Autodesk Inventor part; units mm, degrees
(part 2 of 3)
  line L934 (-2.3825, 17.3276) -> (-2.1489, 17.5795)
  line L935 (-2.1489, 17.5795) -> (-1.9408, 17.8528)
  line L936 (-1.9408, 17.8528) -> (-1.76, 18.1449)
  line L937 (-1.76, 18.1449) -> (-1.6083, 18.4531)
  line L938 (-2.6725, 3.5253) -> (-2.5898, 3.5474)
  line L939 (-16.7895, -16.1624) -> (-16.4169, -16.535)
  line L940 (-15.9078, -14.6352) -> (-16.4089, -14.7796)
  line L941 (15.6533, -16.6714) -> (16.1624, -16.535)
  line L942 (15.502, -16.5103) -> (16.0062, -16.3752)
  line L943 (-2.5898, 3.8338) -> (-2.6725, 3.856)
  line L944 (-2.5648, 3.7968) -> (-2.6467, 3.8187)
  line L945 (-15.0316, -16.1569) -> (-14.8897, -15.6533)
  line L946 (15.1443, -16.535) -> (15.6533, -16.6714)
  line L947 (14.9979, -16.3752) -> (15.502, -16.5103)
  line L948 (14.7716, -16.1624) -> (14.9979, -16.3752)
  line L949 (-12.7709, 17.5782) -> (-12.8535, 17.6003)
  line L950 (-12.6921, 17.4203) -> (-12.7293, 17.4302)
  line L951 (11.4696, 12.9362) -> (11.4091, 12.9967)
  line L952 (4.4542, 16.535) -> (4.0815, 16.1624)
  line L953 (-14.1262, 17.2697) -> (-14.0435, 17.2918)
  line L954 (-2.5293, 3.6079) -> (-2.4935, 3.6943)
  line L955 (-15.3161, -0.4931) -> (-15.3988, -0.471)
  line L956 (-2.7552, 3.5474) -> (-2.6725, 3.5253)
  line L957 (-11.6922, 17.5177) -> (-11.7528, 17.5782)
  line L958 (-12.8535, 17.6003) -> (-12.9362, 17.5782)
  line L959 (-12.7293, 17.4302) -> (-12.8112, 17.4083)
  line L960 (-14.0435, 17.2918) -> (-13.983, 17.3523)
  line L961 (16.535, -16.1624) -> (16.6714, -15.6533)
  line L962 (16.3752, -16.0062) -> (16.5103, -15.502)
  line L963 (16.1624, -16.535) -> (16.535, -16.1624)
  line L964 (16.0062, -16.3752) -> (16.3752, -16.0062)
  line L965 (-16.051, 13.0254) -> (-15.9905, 12.9649)
  line L966 (16.5103, -15.502) -> (16.3752, -14.9979)
  line L967 (10.4801, 13.5058) -> (10.4196, 13.4453)
  line L968 (-12.9362, 17.5782) -> (-12.9967, 17.5177)
  line L969 (-8.8703, 17.435) -> (-8.8925, 17.5177)
  line L970 (16.3752, -14.9979) -> (16.1624, -14.7716)
  line L971 (16.6714, -15.6533) -> (16.535, -15.1443)
  line L972 (-1.0022, 5.6442) -> (-0.985, 5.7255)
  line L973 (-9.1183, 17.5782) -> (-9.1788, 17.5177)
  line L974 (-9.0302, 17.4083) -> (-9.0901, 17.3484)
  line L975 (10.706, 13.2799) -> (10.7282, 13.3626)
  line L976 (14.7784, 2.3353) -> (14.8006, 2.418)
  line L977 (14.6356, 2.3128) -> (14.6575, 2.3946)
  line L978 (10.5628, 13.5279) -> (10.4801, 13.5058)
  line L979 (-13.983, 17.5177) -> (-14.0435, 17.5782)
  line L980 (5.4723, 14.7716) -> (5.8449, 15.1443)
  line L981 (4.9632, 14.6352) -> (5.4723, 14.7716)
  line L982 (16.1699, -9.0744) -> (16.1502, -9.0008)
  line L983 (3.9451, 15.6533) -> (4.0815, 15.1443)
  line L984 (11.1545, -2.0203) -> (11.0719, -1.9981)
  line L985 (4.4542, 14.7716) -> (4.9632, 14.6352)
  line L986 (13.2334, -15.1616) -> (13.3153, -15.1397)
  line L987 (-13.0189, 17.435) -> (-12.9967, 17.3523)
  line L988 (-11.7528, 17.2918) -> (-11.6922, 17.3523)
  line L989 (10.4196, 13.4453) -> (10.3975, 13.3626)
  line L990 (-17.5782, 6.6623) -> (-17.5177, 6.6017)
  line L991 (-8.953, 17.5782) -> (-9.0357, 17.6003)
  line L992 (-8.8767, 17.411) -> (-8.9483, 17.4302)
  line L993 (-2.7885, 3.5731) -> (-2.7552, 3.5474)
  line L994 (16.1624, -14.7716) -> (15.6533, -14.6352)
  line L995 (-11.8354, 17.6003) -> (-11.9181, 17.5782)
  line L996 (-11.721, 17.4302) -> (-11.8029, 17.4083)
  line L997 (5.8449, 16.1624) -> (5.4723, 16.535)
  line L998 (4.0815, 15.1443) -> (4.4542, 14.7716)
  line L999 (5.9813, 15.6533) -> (5.8449, 16.1624)
  line L1000 (-17.2697, 9.2902) -> (-17.2918, 9.3729)
  line L1001 (5.9235, 15.502) -> (5.7885, 16.0062)
  line L1002 (14.7179, 2.2748) -> (14.7784, 2.3353)
  line L1003 (14.5881, 2.2653) -> (14.6356, 2.3128)
  line L1004 (-11.8354, 17.2697) -> (-11.7528, 17.2918)
  line L1005 (-1.0627, 5.5836) -> (-1.0022, 5.6442)
  line L1006 (-17.2918, 9.3729) -> (-17.3523, 9.4334)
  line L1007 (4.9632, 16.6714) -> (4.4542, 16.535)
  line L1008 (15.6533, -14.6352) -> (15.1443, -14.7716)
  line L1009 (-17.6003, 6.7449) -> (-17.5782, 6.6623)
  line L1010 (-1.1454, 5.5615) -> (-1.0627, 5.5836)
  line L1011 (15.1443, -14.7716) -> (14.7716, -15.1443)
  line L1012 (14.7716, -15.1443) -> (14.6352, -15.6533)
  line L1013 (-17.435, 6.9103) -> (-17.5177, 6.8881)
  line L1014 (-9.0357, 17.6003) -> (-9.1183, 17.5782)
  line L1015 (-8.9483, 17.4302) -> (-9.0302, 17.4083)
  line L1016 (-1.228, 5.5836) -> (-1.1454, 5.5615)
  line L1017 (-14.6352, 15.6533) -> (-14.7716, 16.1624)
  line L1018 (-16.1624, 14.7716) -> (-15.6533, 14.6352)
  line L1019 (-16.6714, 15.6533) -> (-16.535, 15.1443)
  line L1020 (-16.535, 16.1624) -> (-16.6714, 15.6533)
  line L1021 (-16.1624, 16.535) -> (-16.535, 16.1624)
  line L1022 (-15.6533, 16.6714) -> (-16.1624, 16.535)
  line L1023 (-15.9078, -16.6714) -> (-15.3988, -16.535)
  line L1024 (-16.4169, -16.535) -> (-15.9078, -16.6714)
  line L1025 (-16.9259, -15.6533) -> (-16.7895, -16.1624)
  line L1026 (-15.3988, -14.7716) -> (-15.9078, -14.6352)
  line L1027 (16.026, -3.4361) -> (16.1624, -2.927)
  line L1028 (15.6533, -3.8087) -> (16.026, -3.4361)
  line L1029 (15.1443, -3.9451) -> (15.6533, -3.8087)
  line L1030 (14.1262, -2.927) -> (14.2626, -3.4361)
  line L1031 (14.2626, -2.418) -> (14.1262, -2.927)
  line L1032 (14.6352, -2.0453) -> (14.2626, -2.418)
  line L1033 (15.6533, -2.0453) -> (15.1443, -1.9089)
  line L1034 (16.026, -2.418) -> (15.6533, -2.0453)
  line L1035 (-13.1081, 15.017) -> (-13.1763, 15.2715)
  line L1036 (-13.1763, 14.7625) -> (-13.1081, 15.017)
  line L1037 (-13.3626, 14.5762) -> (-13.1763, 14.7625)
  line L1038 (-13.6171, 14.508) -> (-13.3626, 14.5762)
  line L1039 (-13.8716, 14.5762) -> (-13.6171, 14.508)
  line L1040 (-14.1262, 15.017) -> (-14.058, 14.7625)
  line L1041 (-14.058, 15.2715) -> (-14.1262, 15.017)
  line L1042 (-13.8716, 15.4579) -> (-14.058, 15.2715)
  line L1043 (-13.6171, 15.5261) -> (-13.8716, 15.4579)
  line L1044 (-13.3626, 15.4579) -> (-13.6171, 15.5261)
  line L1045 (-8.0858, 15.7806) -> (-8.0176, 16.0351)
  line L1046 (-8.2721, 15.5943) -> (-8.0858, 15.7806)
  line L1047 (-8.5266, 15.5261) -> (-8.2721, 15.5943)
  line L1048 (-8.7811, 15.5943) -> (-8.5266, 15.5261)
  line L1049 (-9.0357, 16.0351) -> (-8.9675, 15.7806)
  line L1050 (-8.9675, 16.2896) -> (-9.0357, 16.0351)
  line L1051 (-8.7811, 16.476) -> (-8.9675, 16.2896)
  line L1052 (-8.5266, 16.5442) -> (-8.7811, 16.476)
  line L1053 (-8.2721, 16.476) -> (-8.5266, 16.5442)
  line L1054 (-8.0858, 16.2896) -> (-8.2721, 16.476)
  line L1055 (-8.0858, 13.7444) -> (-8.0176, 13.9989)
  line L1056 (-8.2721, 13.5581) -> (-8.0858, 13.7444)
  line L1057 (-8.7811, 13.5581) -> (-8.5266, 13.4899)
  line L1058 (-8.7811, 14.4398) -> (-8.9675, 14.2534)
  line L1059 (-8.0858, 14.2534) -> (-8.2721, 14.4398)
  line L1060 (-12.5163, 12.9649) -> (-12.4558, 13.0254)
  line L1061 (-12.599, 12.9427) -> (-12.5163, 12.9649)
  line L1062 (-12.7422, 13.0254) -> (-12.6817, 12.9649)
  line L1063 (-12.7644, 13.1081) -> (-12.7422, 13.0254)
  line L1064 (-12.7422, 13.1907) -> (-12.7644, 13.1081)
  line L1065 (-12.6817, 13.2513) -> (-12.7422, 13.1907)
  line L1066 (-12.599, 13.2734) -> (-12.6817, 13.2513)
  line L1067 (-12.5163, 13.2513) -> (-12.599, 13.2734)
  line L1068 (-12.4558, 13.1907) -> (-12.5163, 13.2513)
  line L1069 (-1.228, 5.87) -> (-1.2886, 5.8095)
  line L1070 (-1.1454, 5.8922) -> (-1.228, 5.87)
  line L1071 (-1.0627, 5.87) -> (-1.1454, 5.8922)
  line L1072 (-9.0357, 17.2697) -> (-8.953, 17.2918)
  line L1073 (-9.1183, 17.2918) -> (-9.0357, 17.2697)
  line L1074 (-9.1788, 17.3523) -> (-9.1183, 17.2918)
  line L1075 (11.4917, 12.8535) -> (11.4696, 12.9362)
  line L1076 (11.4091, 12.7103) -> (11.4696, 12.7709)
  line L1077 (11.2437, 12.7103) -> (11.3264, 12.6882)
  line L1078 (11.1832, 12.7709) -> (11.2437, 12.7103)
  line L1079 (11.161, 12.8535) -> (11.1832, 12.7709)
  line L1080 (11.2437, 12.9967) -> (11.1832, 12.9362)
  line L1081 (11.3264, 13.0189) -> (11.2437, 12.9967)
  line L1082 (11.4091, 12.9967) -> (11.3264, 13.0189)
  line L1083 (-11.6922, 17.3523) -> (-11.6701, 17.435)
  line L1084 (-11.9786, 17.5177) -> (-12.0008, 17.435)
  line L1085 (-11.9181, 17.5782) -> (-11.9786, 17.5177)
  line L1086 (10.7282, 13.3626) -> (10.706, 13.4453)
  line L1087 (10.6455, 13.2194) -> (10.706, 13.2799)
  line L1088 (10.4801, 13.2194) -> (10.5628, 13.1972)
  line L1089 (10.4196, 13.2799) -> (10.4801, 13.2194)
  line L1090 (10.3975, 13.3626) -> (10.4196, 13.2799)
  line L1091 (10.706, 13.4453) -> (10.6455, 13.5058)
  line L1092 (8.1829, 15.1443) -> (8.1607, 15.2269)
  line L1093 (8.1607, 15.0616) -> (8.1829, 15.1443)
  line L1094 (8.1002, 15.0011) -> (8.1607, 15.0616)
  line L1095 (8.0176, 14.9789) -> (8.1002, 15.0011)
  line L1096 (7.9349, 15.0011) -> (8.0176, 14.9789)
  line L1097 (7.8744, 15.0616) -> (7.9349, 15.0011)
  line L1098 (7.8522, 15.1443) -> (7.8744, 15.0616)
  line L1099 (7.8744, 15.2269) -> (7.8522, 15.1443)
  line L1100 (7.9349, 15.2875) -> (7.8744, 15.2269)
  line L1101 (8.0176, 15.3096) -> (7.9349, 15.2875)
  line L1102 (8.1002, 15.2875) -> (8.0176, 15.3096)
  line L1103 (8.1607, 15.2269) -> (8.1002, 15.2875)
  line L1104 (-1.2345, 16.4169) -> (-1.2567, 16.4996)
  line L1105 (-1.2477, 16.3432) -> (-1.2345, 16.4169)
  line L1106 (-1.3172, 16.2737) -> (-1.2477, 16.3432)
  line L1107 (-1.3999, 16.2516) -> (-1.3172, 16.2737)
  line L1108 (-1.4826, 16.2737) -> (-1.3999, 16.2516)
  line L1109 (-1.5431, 16.3342) -> (-1.4826, 16.2737)
  line L1110 (-1.5652, 16.4169) -> (-1.5431, 16.3342)
  line L1111 (-1.5431, 16.4996) -> (-1.5652, 16.4169)
  line L1112 (-1.4826, 16.5601) -> (-1.5431, 16.4996)
  line L1113 (-1.3999, 16.5822) -> (-1.4826, 16.5601)
  line L1114 (-1.3172, 16.5601) -> (-1.3999, 16.5822)
  line L1115 (-1.2567, 16.4996) -> (-1.3172, 16.5601)
  line L1116 (10.7282, 15.3988) -> (10.706, 15.4815)
  line L1117 (10.706, 15.4815) -> (10.6455, 15.542)
  line L1118 (14.546, -12.599) -> (14.5239, -12.5163)
  line L1119 (14.5239, -12.6817) -> (14.546, -12.599)
  line L1120 (14.4634, -12.7422) -> (14.5239, -12.6817)
  line L1121 (14.3807, -12.7644) -> (14.4634, -12.7422)
  line L1122 (14.298, -12.7422) -> (14.3807, -12.7644)
  line L1123 (14.2375, -12.6817) -> (14.298, -12.7422)
  line L1124 (14.2375, -12.5163) -> (14.2154, -12.599)
  line L1125 (14.298, -12.4558) -> (14.2375, -12.5163)
  line L1126 (14.3807, -12.4337) -> (14.298, -12.4558)
  line L1127 (14.4634, -12.4558) -> (14.3807, -12.4337)
  line L1128 (14.5239, -12.5163) -> (14.4634, -12.4558)
  line L1129 (6.6557, -17.435) -> (6.6336, -17.3523)
  line L1130 (6.6336, -17.5177) -> (6.6557, -17.435)
  line L1131 (6.5731, -17.5782) -> (6.6336, -17.5177)
  line L1132 (6.4904, -17.6003) -> (6.5731, -17.5782)
  line L1133 (6.4077, -17.5782) -> (6.4904, -17.6003)
  line L1134 (6.3472, -17.5177) -> (6.4077, -17.5782)
  line L1135 (6.3251, -17.435) -> (6.3472, -17.5177)
  line L1136 (6.4077, -17.2918) -> (6.3472, -17.3523)
  line L1137 (6.4904, -17.2697) -> (6.4077, -17.2918)
  line L1138 (6.5731, -17.2918) -> (6.4904, -17.2697)
  line L1139 (6.6336, -17.3523) -> (6.5731, -17.2918)
  line L1140 (0.0381, -17.435) -> (0.0159, -17.3523)
  line L1141 (0.0159, -17.5177) -> (0.0381, -17.435)
  line L1142 (-0.0446, -17.5782) -> (0.0159, -17.5177)
  line L1143 (-0.1273, -17.6003) -> (-0.0446, -17.5782)
  line L1144 (-0.2099, -17.5782) -> (-0.1273, -17.6003)
  line L1145 (-0.2705, -17.5177) -> (-0.2099, -17.5782)
  line L1146 (-0.2099, -17.2918) -> (-0.2705, -17.3523)
  line L1147 (-0.1273, -17.2697) -> (-0.2099, -17.2918)
  line L1148 (-0.0446, -17.2918) -> (-0.1273, -17.2697)
  line L1149 (0.0159, -17.3523) -> (-0.0446, -17.2918)
  line L1150 (-5.8382, -15.736) -> (-5.816, -15.6533)
  line L1151 (-5.8987, -15.7965) -> (-5.8382, -15.736)
  line L1152 (-5.9813, -15.8187) -> (-5.8987, -15.7965)
  line L1153 (-6.064, -15.7965) -> (-5.9813, -15.8187)
  line L1154 (-6.1245, -15.736) -> (-6.064, -15.7965)
  line L1155 (-6.1467, -15.6533) -> (-6.1245, -15.736)
  line L1156 (-6.1245, -15.5706) -> (-6.1467, -15.6533)
  line L1157 (-5.9813, -15.488) -> (-6.064, -15.5101)
  line L1158 (-5.8987, -15.5101) -> (-5.9813, -15.488)
  line L1159 (-5.8382, -15.5706) -> (-5.8987, -15.5101)
  line L1160 (-8.8703, -14.8897) -> (-8.8925, -14.8071)
  line L1161 (-8.8925, -14.9724) -> (-8.8703, -14.8897)
  line L1162 (-8.953, -15.0329) -> (-8.8925, -14.9724)
  line L1163 (-9.0357, -15.0551) -> (-8.953, -15.0329)
  line L1164 (-9.1183, -15.0329) -> (-9.0357, -15.0551)
  line L1165 (-9.1788, -14.9724) -> (-9.1183, -15.0329)
  line L1166 (-9.201, -14.8897) -> (-9.1788, -14.9724)
  line L1167 (-9.1788, -14.8071) -> (-9.201, -14.8897)
  line L1168 (-9.1183, -14.7466) -> (-9.1788, -14.8071)
  line L1169 (-9.0357, -14.7244) -> (-9.1183, -14.7466)
  line L1170 (-8.953, -14.7466) -> (-9.0357, -14.7244)
  line L1171 (-8.8925, -14.8071) -> (-8.953, -14.7466)
  line L1172 (-11.6701, -14.8897) -> (-11.6922, -14.8071)
  line L1173 (-11.6922, -14.9724) -> (-11.6701, -14.8897)
  line L1174 (-11.7528, -15.0329) -> (-11.6922, -14.9724)
  line L1175 (-11.8354, -15.0551) -> (-11.7528, -15.0329)
  line L1176 (-11.9181, -15.0329) -> (-11.8354, -15.0551)
  line L1177 (-11.9786, -14.9724) -> (-11.9181, -15.0329)
  line L1178 (-12.0008, -14.8897) -> (-11.9786, -14.9724)
  line L1179 (-11.9786, -14.8071) -> (-12.0008, -14.8897)
  line L1180 (-11.9181, -14.7466) -> (-11.9786, -14.8071)
  line L1181 (-11.7528, -14.7466) -> (-11.8354, -14.7244)
  line L1182 (-11.6922, -14.8071) -> (-11.7528, -14.7466)
  line L1183 (-13.4518, -15.9078) -> (-13.4739, -15.8252)
  line L1184 (-13.4739, -15.9905) -> (-13.4518, -15.9078)
  line L1185 (-13.5344, -16.051) -> (-13.4739, -15.9905)
  line L1186 (-13.6171, -16.0732) -> (-13.5344, -16.051)
  line L1187 (-13.6998, -16.051) -> (-13.6171, -16.0732)
  line L1188 (-13.7603, -15.9905) -> (-13.6998, -16.051)
  line L1189 (-13.7825, -15.9078) -> (-13.7603, -15.9905)
  line L1190 (-13.7603, -15.8252) -> (-13.7825, -15.9078)
  line L1191 (-13.6998, -15.7647) -> (-13.7603, -15.8252)
  line L1192 (-13.5344, -15.7647) -> (-13.6171, -15.7425)
  line L1193 (-13.4739, -15.8252) -> (-13.5344, -15.7647)
  line L1194 (-15.0011, -17.3904) -> (-14.9789, -17.3077)
  line L1195 (-15.0616, -17.4509) -> (-15.0011, -17.3904)
  line L1196 (-15.1443, -17.4731) -> (-15.0616, -17.4509)
  line L1197 (-15.2269, -17.4509) -> (-15.1443, -17.4731)
  line L1198 (-15.2875, -17.3904) -> (-15.2269, -17.4509)
  line L1199 (-15.3096, -17.3077) -> (-15.2875, -17.3904)
  line L1200 (-15.2875, -17.2251) -> (-15.3096, -17.3077)
  line L1201 (-15.2269, -17.1645) -> (-15.2875, -17.2251)
  line L1202 (-15.1443, -17.1424) -> (-15.2269, -17.1645)
  line L1203 (-15.0616, -17.1645) -> (-15.1443, -17.1424)
  line L1204 (-15.0011, -17.2251) -> (-15.0616, -17.1645)
  line L1205 (-17.2697, -14.7625) -> (-17.2918, -14.6798)
  line L1206 (-17.3523, -14.9057) -> (-17.2918, -14.8452)
  line L1207 (-17.435, -14.9278) -> (-17.3523, -14.9057)
  line L1208 (-17.5177, -14.9057) -> (-17.435, -14.9278)
  line L1209 (-17.5782, -14.8452) -> (-17.5177, -14.9057)
  line L1210 (-17.6003, -14.7625) -> (-17.5782, -14.8452)
  line L1211 (-17.5782, -14.6798) -> (-17.6003, -14.7625)
  line L1212 (-17.5177, -14.6193) -> (-17.5782, -14.6798)
  line L1213 (-17.435, -14.5971) -> (-17.5177, -14.6193)
  line L1214 (-17.3523, -14.6193) -> (-17.435, -14.5971)
  line L1215 (-17.2918, -14.6798) -> (-17.3523, -14.6193)
  line L1216 (-15.488, -13.3626) -> (-15.5101, -13.2799)
  line L1217 (-15.5706, -13.5058) -> (-15.5101, -13.4453)
  line L1218 (-15.6533, -13.5279) -> (-15.5706, -13.5058)
  line L1219 (-15.736, -13.5058) -> (-15.6533, -13.5279)
  line L1220 (-15.7965, -13.4453) -> (-15.736, -13.5058)
  line L1221 (-15.8187, -13.3626) -> (-15.7965, -13.4453)
  line L1222 (-15.7965, -13.2799) -> (-15.8187, -13.3626)
  line L1223 (-15.736, -13.2194) -> (-15.7965, -13.2799)
  line L1224 (-15.6533, -13.1972) -> (-15.736, -13.2194)
  line L1225 (-15.5706, -13.2194) -> (-15.6533, -13.1972)
  line L1226 (-15.5101, -13.2799) -> (-15.5706, -13.2194)
  line L1227 (-14.9789, -11.5809) -> (-15.0011, -11.4982)
  line L1228 (-15.0616, -11.7241) -> (-15.0011, -11.6636)
  line L1229 (-15.1443, -11.7463) -> (-15.0616, -11.7241)
  line L1230 (-15.2269, -11.7241) -> (-15.1443, -11.7463)
  line L1231 (-15.2875, -11.6636) -> (-15.2269, -11.7241)
  line L1232 (-15.3096, -11.5809) -> (-15.2875, -11.6636)
  line L1233 (-15.2875, -11.4982) -> (-15.3096, -11.5809)
  line L1234 (-15.2269, -11.4377) -> (-15.2875, -11.4982)
  line L1235 (-15.1443, -11.4156) -> (-15.2269, -11.4377)
  line L1236 (-15.0616, -11.4377) -> (-15.1443, -11.4156)
  line L1237 (-15.0011, -11.4982) -> (-15.0616, -11.4377)
  line L1238 (-14.7244, -8.7811) -> (-14.7466, -8.6985)
  line L1239 (-14.7466, -8.8638) -> (-14.7244, -8.7811)
  line L1240 (-14.8071, -8.9243) -> (-14.7466, -8.8638)
  line L1241 (-14.8897, -8.9465) -> (-14.8071, -8.9243)
  line L1242 (-14.9724, -8.9243) -> (-14.8897, -8.9465)
  line L1243 (-15.0329, -8.8638) -> (-14.9724, -8.9243)
  line L1244 (-15.0551, -8.7811) -> (-15.0329, -8.8638)
  line L1245 (-15.0329, -8.6985) -> (-15.0551, -8.7811)
  line L1246 (-14.9724, -8.6379) -> (-15.0329, -8.6985)
  line L1247 (-14.8897, -8.6158) -> (-14.9724, -8.6379)
  line L1248 (-14.8071, -8.6379) -> (-14.8897, -8.6158)
  line L1249 (-14.7466, -8.6985) -> (-14.8071, -8.6379)
  line L1250 (-15.488, -6.2359) -> (-15.5101, -6.1532)
  line L1251 (-15.5101, -6.3185) -> (-15.488, -6.2359)
  line L1252 (-15.5706, -6.3791) -> (-15.5101, -6.3185)
  line L1253 (-15.6533, -6.4012) -> (-15.5706, -6.3791)
  line L1254 (-15.736, -6.3791) -> (-15.6533, -6.4012)
  line L1255 (-15.7965, -6.3185) -> (-15.736, -6.3791)
  line L1256 (-15.8187, -6.2359) -> (-15.7965, -6.3185)
  line L1257 (-15.7965, -6.1532) -> (-15.8187, -6.2359)
  line L1258 (-15.736, -6.0927) -> (-15.7965, -6.1532)
  line L1259 (-15.6533, -6.0705) -> (-15.736, -6.0927)
  line L1260 (-15.5101, -6.1532) -> (-15.5706, -6.0927)
  line L1261 (-17.2697, -4.1997) -> (-17.2918, -4.117)
  line L1262 (-17.2918, -4.2823) -> (-17.2697, -4.1997)
  line L1263 (-17.435, -4.365) -> (-17.3523, -4.3429)
  line L1264 (-17.5177, -4.3429) -> (-17.435, -4.365)
  line L1265 (-17.5782, -4.2823) -> (-17.5177, -4.3429)
  line L1266 (-17.6003, -4.1997) -> (-17.5782, -4.2823)
  line L1267 (-17.5782, -4.117) -> (-17.6003, -4.1997)
  line L1268 (-17.5177, -4.0565) -> (-17.5782, -4.117)
  line L1269 (-17.435, -4.0343) -> (-17.5177, -4.0565)
  line L1270 (-17.2918, -4.117) -> (-17.3523, -4.0565)
  line L1271 (-17.2697, -1.6544) -> (-17.2918, -1.5717)
  line L1272 (-17.2918, -1.7371) -> (-17.2697, -1.6544)
  line L1273 (-17.3523, -1.7976) -> (-17.2918, -1.7371)
  line L1274 (-17.435, -1.8198) -> (-17.3523, -1.7976)
  line L1275 (-17.5177, -1.7976) -> (-17.435, -1.8198)
  line L1276 (-17.5782, -1.7371) -> (-17.5177, -1.7976)
  line L1277 (-17.6003, -1.6544) -> (-17.5782, -1.7371)
  line L1278 (-17.5782, -1.5717) -> (-17.6003, -1.6544)
  line L1279 (-17.5177, -1.5112) -> (-17.5782, -1.5717)
  line L1280 (-17.435, -1.4891) -> (-17.5177, -1.5112)
  line L1281 (-17.3523, -1.5112) -> (-17.435, -1.4891)
  line L1282 (-17.2918, -1.5717) -> (-17.3523, -1.5112)
  line L1283 (-17.2697, 0.8908) -> (-17.2918, 0.9735)
  line L1284 (-17.2918, 0.8082) -> (-17.2697, 0.8908)
  line L1285 (-17.3523, 0.7476) -> (-17.2918, 0.8082)
  line L1286 (-17.435, 0.7255) -> (-17.3523, 0.7476)
  line L1287 (-17.5177, 0.7476) -> (-17.435, 0.7255)
  line L1288 (-17.5782, 0.8082) -> (-17.5177, 0.7476)
  line L1289 (-17.6003, 0.8908) -> (-17.5782, 0.8082)
  line L1290 (-17.5782, 0.9735) -> (-17.6003, 0.8908)
  line L1291 (-17.5177, 1.034) -> (-17.5782, 0.9735)
  line L1292 (-17.435, 1.0562) -> (-17.5177, 1.034)
  line L1293 (-17.3523, 1.034) -> (-17.435, 1.0562)
  line L1294 (-17.2918, 0.9735) -> (-17.3523, 1.034)
  line L1295 (-17.2697, 3.6906) -> (-17.2918, 3.7733)
  line L1296 (-17.2918, 3.6079) -> (-17.2697, 3.6906)
  line L1297 (-17.3523, 3.5474) -> (-17.2918, 3.6079)
  line L1298 (-17.5177, 3.5474) -> (-17.435, 3.5253)
  line L1299 (-17.5782, 3.6079) -> (-17.5177, 3.5474)
  line L1300 (-17.6003, 3.6906) -> (-17.5782, 3.6079)
  line L1301 (-17.5782, 3.7733) -> (-17.6003, 3.6906)
  line L1302 (-17.5177, 3.8338) -> (-17.5782, 3.7733)
  line L1303 (-17.435, 3.856) -> (-17.5177, 3.8338)
  line L1304 (-17.3523, 3.8338) -> (-17.435, 3.856)
  line L1305 (-17.2697, 6.7449) -> (-17.2918, 6.8276)
  line L1306 (-17.2918, 6.6623) -> (-17.2697, 6.7449)
  line L1307 (-17.3523, 6.6017) -> (-17.2918, 6.6623)
  line L1308 (-17.5177, 6.6017) -> (-17.435, 6.5796)
  line L1309 (-17.5782, 6.8276) -> (-17.6003, 6.7449)
  line L1310 (-17.5177, 6.8881) -> (-17.5782, 6.8276)
  line L1311 (-17.3523, 6.8881) -> (-17.435, 6.9103)
  line L1312 (-17.2918, 6.8276) -> (-17.3523, 6.8881)
  line L1313 (-17.2918, 9.2075) -> (-17.2697, 9.2902)
  line L1314 (-17.3523, 9.147) -> (-17.2918, 9.2075)
  line L1315 (-17.5177, 9.147) -> (-17.435, 9.1248)
  line L1316 (-17.5782, 9.2075) -> (-17.5177, 9.147)
  line L1317 (-17.6003, 9.2902) -> (-17.5782, 9.2075)
  line L1318 (-17.5782, 9.3729) -> (-17.6003, 9.2902)
  line L1319 (-17.5177, 9.4334) -> (-17.5782, 9.3729)
  line L1320 (-17.435, 9.4555) -> (-17.5177, 9.4334)
  line L1321 (-17.2918, 11.4982) -> (-17.2697, 11.5809)
  line L1322 (-17.3523, 11.4377) -> (-17.2918, 11.4982)
  line L1323 (-17.435, 11.4156) -> (-17.3523, 11.4377)
  line L1324 (-17.5177, 11.4377) -> (-17.435, 11.4156)
  line L1325 (-17.5782, 11.4982) -> (-17.5177, 11.4377)
  line L1326 (-17.6003, 11.5809) -> (-17.5782, 11.4982)
  line L1327 (-17.5782, 11.6636) -> (-17.6003, 11.5809)
  line L1328 (-17.5177, 11.7241) -> (-17.5782, 11.6636)
  line L1329 (-17.435, 11.7463) -> (-17.5177, 11.7241)
  line L1330 (-17.3523, 11.7241) -> (-17.435, 11.7463)
  line L1331 (-17.2918, 11.6636) -> (-17.3523, 11.7241)
  line L1332 (-17.0373, 12.7709) -> (-17.0151, 12.8535)
  line L1333 (-17.0978, 12.7103) -> (-17.0373, 12.7709)
  line L1334 (-17.168, 12.6915) -> (-17.0978, 12.7103)
  line L1335 (-17.2631, 12.7103) -> (-17.168, 12.6915)
  line L1336 (-17.3237, 12.7709) -> (-17.2631, 12.7103)
  line L1337 (-17.2631, 12.9967) -> (-17.3237, 12.9362)
  line L1338 (-15.7647, 13.0254) -> (-15.7425, 13.1081)
  line L1339 (-15.8252, 12.9649) -> (-15.7647, 13.0254)
  line L1340 (-15.9078, 12.9427) -> (-15.8252, 12.9649)
  line L1341 (-15.9905, 12.9649) -> (-15.9078, 12.9427)
  line L1342 (-16.0732, 13.1081) -> (-16.051, 13.0254)
  line L1343 (-15.9078, 13.2734) -> (-15.9905, 13.2513)
  line L1344 (-15.8252, 13.2513) -> (-15.9078, 13.2734)
  line L1345 (-15.7647, 13.1907) -> (-15.8252, 13.2513)
  line L1346 (-13.9608, 17.435) -> (-13.983, 17.5177)
  line L1347 (-13.983, 17.3523) -> (-13.9608, 17.435)
  line L1348 (-14.2694, 17.3523) -> (-14.2088, 17.2918)
  line L1349 (-14.2915, 17.435) -> (-14.2694, 17.3523)
  line L1350 (-14.2088, 17.5782) -> (-14.2694, 17.5177)
  line L1351 (-14.0435, 17.5782) -> (-14.1262, 17.6003)
  line L1352 (-12.6921, 17.4203) -> (-12.7103, 17.5177)
  line L1353 (-12.7103, 17.3523) -> (-12.6921, 17.4203)
  line L1354 (-12.7709, 17.2918) -> (-12.7103, 17.3523)
  line L1355 (-12.8535, 17.2697) -> (-12.7709, 17.2918)
  line L1356 (-12.9967, 17.3523) -> (-12.9362, 17.2918)
  line L1357 (-12.9967, 17.5177) -> (-13.0189, 17.435)
  line L1358 (-12.7103, 17.5177) -> (-12.7709, 17.5782)
  line L1359 (-16.2516, 5.4723) -> (-16.2737, 5.555)
  line L1360 (-16.2737, 5.3896) -> (-16.2516, 5.4723)
  line L1361 (-16.3342, 5.3291) -> (-16.2737, 5.3896)
  line L1362 (-16.4996, 5.3291) -> (-16.4169, 5.307)
  line L1363 (-16.5601, 5.3896) -> (-16.4996, 5.3291)
  line L1364 (-16.5822, 5.4723) -> (-16.5601, 5.3896)
  line L1365 (-16.5601, 5.555) -> (-16.5822, 5.4723)
  line L1366 (-16.4996, 5.6155) -> (-16.5601, 5.555)
  line L1367 (-16.4169, 5.6376) -> (-16.4996, 5.6155)
  line L1368 (-16.3342, 5.6155) -> (-16.4169, 5.6376)
  line L1369 (-16.0192, 11.7528) -> (-15.997, 11.8354)
  line L1370 (-16.0797, 11.6922) -> (-16.0192, 11.7528)
  line L1371 (-16.1624, 11.6701) -> (-16.0797, 11.6922)
  line L1372 (-16.245, 11.6922) -> (-16.1624, 11.6701)
  line L1373 (-16.3056, 11.7528) -> (-16.245, 11.6922)
  line L1374 (-16.3277, 11.8354) -> (-16.3056, 11.7528)
  line L1375 (-16.3056, 11.9181) -> (-16.3277, 11.8354)
  line L1376 (-16.245, 11.9786) -> (-16.3056, 11.9181)
  line L1377 (-16.1624, 12.0008) -> (-16.245, 11.9786)
  line L1378 (-16.0797, 11.9786) -> (-16.1624, 12.0008)
  line L1379 (-16.0192, 11.9181) -> (-16.0797, 11.9786)
  line L1380 (-6.3472, 14.1708) -> (-6.3251, 14.2534)
  line L1381 (-6.4077, 14.1102) -> (-6.3472, 14.1708)
  line L1382 (-6.4904, 14.0881) -> (-6.4077, 14.1102)
  line L1383 (-6.3472, 14.3361) -> (-6.4077, 14.3966)
  line L1384 (-5.3291, 13.9162) -> (-5.307, 13.9989)
  line L1385 (-5.3896, 13.8557) -> (-5.3291, 13.9162)
  line L1386 (-5.4723, 13.8336) -> (-5.3896, 13.8557)
  line L1387 (-5.555, 13.8557) -> (-5.4723, 13.8336)
  line L1388 (-5.6376, 13.9989) -> (-5.6155, 13.9162)
  line L1389 (-5.6155, 14.0816) -> (-5.6376, 13.9989)
  line L1390 (-5.555, 14.1421) -> (-5.6155, 14.0816)
  line L1391 (-5.4723, 14.1642) -> (-5.555, 14.1421)
  line L1392 (-0.9735, 17.2918) -> (-0.8908, 17.2697)
  line L1393 (1.0562, 17.435) -> (1.034, 17.5177)
  line L1394 (1.034, 17.3523) -> (1.0562, 17.435)
  line L1395 (0.9735, 17.2918) -> (1.034, 17.3523)
  line L1396 (0.8908, 17.2697) -> (0.9735, 17.2918)
  line L1397 (0.8082, 17.2918) -> (0.8908, 17.2697)
  line L1398 (0.7476, 17.3523) -> (0.8082, 17.2918)
  line L1399 (0.7255, 17.435) -> (0.7476, 17.3523)
  line L1400 (0.7476, 17.5177) -> (0.7255, 17.435)
  line L1401 (0.8082, 17.5782) -> (0.7476, 17.5177)
  line L1402 (0.8908, 17.6003) -> (0.8082, 17.5782)
  line L1403 (0.9735, 17.5782) -> (0.8908, 17.6003)
  line L1404 (1.034, 17.5177) -> (0.9735, 17.5782)
  line L1405 (7.6738, 16.6714) -> (7.6517, 16.7541)
  line L1406 (7.6517, 16.5888) -> (7.6738, 16.6714)
  line L1407 (7.5912, 16.5282) -> (7.6517, 16.5888)
  line L1408 (7.5085, 16.5061) -> (7.5912, 16.5282)
  line L1409 (7.4258, 16.5282) -> (7.5085, 16.5061)
  line L1410 (7.3653, 16.5888) -> (7.4258, 16.5282)
  line L1411 (7.3653, 16.7541) -> (7.3432, 16.6714)
  line L1412 (7.4258, 16.8146) -> (7.3653, 16.7541)
  line L1413 (7.5085, 16.8368) -> (7.4258, 16.8146)
  line L1414 (7.5912, 16.8146) -> (7.5085, 16.8368)
  line L1415 (7.6517, 16.7541) -> (7.5912, 16.8146)
  line L1416 (3.3248, 15.3161) -> (3.3469, 15.3988)
  line L1417 (3.1816, 15.2335) -> (3.2642, 15.2556)
  line L1418 (3.3248, 15.4815) -> (3.2642, 15.542)
  line L1419 (15.2556, 10.4801) -> (15.3161, 10.4196)
  line L1420 (15.3988, 10.7282) -> (15.3161, 10.706)
  line L1421 (15.4815, 10.706) -> (15.3988, 10.7282)
  line L1422 (14.546, 9.7992) -> (14.5239, 9.8819)
  line L1423 (14.5239, 9.7166) -> (14.546, 9.7992)
  line L1424 (14.4634, 9.656) -> (14.5239, 9.7166)
  line L1425 (14.3807, 9.6339) -> (14.4634, 9.656)
  line L1426 (14.298, 9.656) -> (14.3807, 9.6339)
  line L1427 (14.2375, 9.7166) -> (14.298, 9.656)
  line L1428 (14.2154, 9.7992) -> (14.2375, 9.7166)
  line L1429 (14.2375, 9.8819) -> (14.2154, 9.7992)
  line L1430 (14.298, 9.9424) -> (14.2375, 9.8819)
  line L1431 (14.3807, 9.9646) -> (14.298, 9.9424)
  line L1432 (14.4634, 9.9424) -> (14.3807, 9.9646)
  line L1433 (14.5239, 9.8819) -> (14.4634, 9.9424)
  line L1434 (14.2694, 3.6079) -> (14.2915, 3.6906)
  line L1435 (14.2088, 3.5474) -> (14.2694, 3.6079)
  line L1436 (14.1262, 3.5253) -> (14.2088, 3.5474)
  line L1437 (13.983, 3.6079) -> (14.0435, 3.5474)
  line L1438 (13.9608, 3.6906) -> (13.983, 3.6079)
  line L1439 (13.983, 3.7733) -> (13.9608, 3.6906)
  line L1440 (14.1262, 3.856) -> (14.0435, 3.8338)
  line L1441 (14.2088, 3.8338) -> (14.1262, 3.856)
  line L1442 (14.2694, 3.7733) -> (14.2088, 3.8338)
  line L1443 (12.7422, 2.9716) -> (12.7644, 3.0543)
  line L1444 (12.6817, 2.9111) -> (12.7422, 2.9716)
  line L1445 (12.4337, 3.0543) -> (12.4558, 2.9716)
  line L1446 (12.4558, 3.137) -> (12.4337, 3.0543)
  line L1447 (12.6817, 3.1975) -> (12.599, 3.2196)
  line L1448 (17.5782, -0.8462) -> (17.6003, -0.7636)
  line L1449 (17.5177, -0.9068) -> (17.5782, -0.8462)
  line L1450 (17.435, -0.9289) -> (17.5177, -0.9068)
  line L1451 (16.3056, -0.719) -> (16.3277, -0.6363)
  line L1452 (16.245, -0.7795) -> (16.3056, -0.719)
  line L1453 (16.1624, -0.8017) -> (16.245, -0.7795)
  line L1454 (16.0797, -0.7795) -> (16.1624, -0.8017)
  line L1455 (16.3056, -0.5536) -> (16.245, -0.4931)
  line L1456 (13.7825, -5.9813) -> (13.7603, -5.8987)
  line L1457 (13.7603, -6.064) -> (13.7825, -5.9813)
  line L1458 (13.6998, -6.1245) -> (13.7603, -6.064)
  line L1459 (13.6171, -6.1467) -> (13.6998, -6.1245)
  line L1460 (13.5344, -6.1245) -> (13.6171, -6.1467)
  line L1461 (13.4518, -5.9813) -> (13.4739, -6.064)
  line L1462 (13.4739, -5.8987) -> (13.4518, -5.9813)
  line L1463 (13.5344, -5.8382) -> (13.4739, -5.8987)
  line L1464 (13.6171, -5.816) -> (13.5344, -5.8382)
  line L1465 (13.6998, -5.8382) -> (13.6171, -5.816)
  line L1466 (13.7603, -5.8987) -> (13.6998, -5.8382)
  line L1467 (14.2915, -8.0176) -> (14.2694, -7.9349)
  line L1468 (14.2088, -7.8744) -> (14.1262, -7.8522)
  line L1469 (14.2694, -7.9349) -> (14.2088, -7.8744)
  line L1470 (8.8192, -13.8716) -> (8.7971, -13.789)
  line L1471 (8.7971, -13.9543) -> (8.8192, -13.8716)
  line L1472 (8.7365, -14.0148) -> (8.7971, -13.9543)
  line L1473 (8.6539, -14.037) -> (8.7365, -14.0148)
  line L1474 (8.5712, -14.0148) -> (8.6539, -14.037)
  line L1475 (8.5107, -13.9543) -> (8.5712, -14.0148)
  line L1476 (8.4884, -13.8794) -> (8.5107, -13.9543)
  line L1477 (8.5107, -13.789) -> (8.4884, -13.8794)
  line L1478 (8.5712, -13.7285) -> (8.5107, -13.789)
  line L1479 (8.6539, -13.7063) -> (8.5712, -13.7285)
  line L1480 (8.734, -13.7376) -> (8.6539, -13.7063)
  line L1481 (8.7971, -13.789) -> (8.734, -13.7376)
  line L1482 (-2.3353, 14.6193) -> (-2.2748, 14.6798)
  line L1483 (4.9792, -14.4634) -> (5.0013, -14.3807)
  line L1484 (4.9187, -14.5239) -> (4.9792, -14.4634)
  line L1485 (4.836, -14.546) -> (4.9187, -14.5239)
  line L1486 (4.7533, -14.5239) -> (4.836, -14.546)
  line L1487 (4.6928, -14.4634) -> (4.7533, -14.5239)
  line L1488 (4.6706, -14.3807) -> (4.6928, -14.4634)
  line L1489 (4.7533, -14.2375) -> (4.6928, -14.298)
  line L1490 (4.836, -14.2154) -> (4.7533, -14.2375)
  line L1491 (4.9187, -14.2375) -> (4.836, -14.2154)
  line L1492 (-0.7255, -15.3988) -> (-0.7476, -15.3161)
  line L1493 (-0.7476, -15.4815) -> (-0.7255, -15.3988)
  line L1494 (-0.8082, -15.542) -> (-0.7476, -15.4815)
  line L1495 (-0.8908, -15.5641) -> (-0.8082, -15.542)
  line L1496 (-0.9735, -15.542) -> (-0.8908, -15.5641)
  line L1497 (-1.034, -15.4815) -> (-0.9735, -15.542)
  line L1498 (-1.0562, -15.3988) -> (-1.034, -15.4815)
  line L1499 (-1.034, -15.3161) -> (-1.0562, -15.3988)
  line L1500 (-0.9735, -15.2556) -> (-1.034, -15.3161)
  line L1501 (-0.8908, -15.2335) -> (-0.9735, -15.2556)
  line L1502 (-0.8082, -15.2556) -> (-0.8908, -15.2335)
  line L1503 (-0.7476, -15.3161) -> (-0.8082, -15.2556)
  line L1504 (-13.3245, -13.4899) -> (-13.3467, -13.4072)
  line L1505 (-13.4072, -13.633) -> (-13.3467, -13.5725)
  line L1506 (-13.4899, -13.6552) -> (-13.4072, -13.633)
  line L1507 (-13.5725, -13.633) -> (-13.4899, -13.6552)
  line L1508 (-13.633, -13.5725) -> (-13.5725, -13.633)
  line L1509 (-13.6552, -13.4899) -> (-13.633, -13.5725)
  line L1510 (-13.633, -13.4072) -> (-13.6552, -13.4899)
  line L1511 (-13.5725, -13.3467) -> (-13.633, -13.4072)
  line L1512 (-13.4072, -13.3467) -> (-13.4899, -13.3245)
  line L1513 (-13.0921, 10.4801) -> (-13.07, 10.5628)
  line L1514 (-13.2529, 10.3927) -> (-13.1527, 10.4196)
  line L1515 (-13.318, 10.4196) -> (-13.2529, 10.3927)
  line L1516 (-13.2353, 10.7282) -> (-13.318, 10.706)
  line L1517 (-13.1527, 10.706) -> (-13.2353, 10.7282)
  line L1518 (-13.0921, 10.6455) -> (-13.1527, 10.706)
  line L1519 (-11.1832, 12.7709) -> (-11.161, 12.8535)
  line L1520 (-11.2437, 12.7103) -> (-11.1832, 12.7709)
  line L1521 (-11.3264, 12.6882) -> (-11.2437, 12.7103)
  line L1522 (-11.4696, 12.7709) -> (-11.4091, 12.7103)
  line L1523 (-11.4917, 12.8535) -> (-11.4696, 12.7709)
  line L1524 (-11.4696, 12.9362) -> (-11.4917, 12.8535)
  line L1525 (-11.4091, 12.9967) -> (-11.4696, 12.9362)
  line L1526 (-11.3264, 13.0189) -> (-11.4091, 12.9967)
  line L1527 (-11.2437, 12.9967) -> (-11.3264, 13.0189)
  line L1528 (-11.1832, 12.9362) -> (-11.2437, 12.9967)
  line L1529 (-14.2375, 13.2799) -> (-14.2154, 13.3626)
  line L1530 (-14.298, 13.2194) -> (-14.2375, 13.2799)
  line L1531 (-14.3807, 13.1972) -> (-14.298, 13.2194)
  line L1532 (-14.4634, 13.2194) -> (-14.3807, 13.1972)
  line L1533 (-14.5239, 13.2799) -> (-14.4634, 13.2194)
  line L1534 (-14.546, 13.3626) -> (-14.5239, 13.2799)
  line L1535 (-14.5239, 13.4453) -> (-14.546, 13.3626)
  line L1536 (-14.4634, 13.5058) -> (-14.5239, 13.4453)
  line L1537 (-14.3807, 13.5279) -> (-14.4634, 13.5058)
  line L1538 (-14.298, 13.5058) -> (-14.3807, 13.5279)
  line L1539 (-14.2375, 13.4453) -> (-14.298, 13.5058)
  line L1540 (-14.8738, 11.4982) -> (-14.8517, 11.5809)
  line L1541 (-14.9343, 11.4377) -> (-14.8738, 11.4982)
  line L1542 (-15.017, 11.4156) -> (-14.9343, 11.4377)
  line L1543 (-15.0997, 11.4377) -> (-15.017, 11.4156)
  line L1544 (-15.1602, 11.4982) -> (-15.0997, 11.4377)
  line L1545 (-15.1823, 11.5809) -> (-15.1602, 11.4982)
  line L1546 (-15.1602, 11.6636) -> (-15.1823, 11.5809)
  line L1547 (-15.0997, 11.7241) -> (-15.1602, 11.6636)
  line L1548 (-15.017, 11.7463) -> (-15.0997, 11.7241)
  line L1549 (-14.9343, 11.7241) -> (-15.017, 11.7463)
  line L1550 (-14.8738, 11.6636) -> (-14.9343, 11.7241)
  line L1551 (-14.8517, 9.2902) -> (-14.8738, 9.3729)
  line L1552 (-14.8738, 9.2075) -> (-14.8517, 9.2902)
  line L1553 (-14.9343, 9.147) -> (-14.8738, 9.2075)
  line L1554 (-15.017, 9.1248) -> (-14.9343, 9.147)
  line L1555 (-15.0997, 9.147) -> (-15.017, 9.1248)
  line L1556 (-15.1602, 9.2075) -> (-15.0997, 9.147)
  line L1557 (-15.1823, 9.2902) -> (-15.1602, 9.2075)
  line L1558 (-15.1602, 9.3729) -> (-15.1823, 9.2902)
  line L1559 (-15.0997, 9.4334) -> (-15.1602, 9.3729)
  line L1560 (-15.017, 9.4555) -> (-15.0997, 9.4334)
  line L1561 (-14.9343, 9.4334) -> (-15.017, 9.4555)
  line L1562 (-14.8738, 9.3729) -> (-14.9343, 9.4334)
  line L1563 (17.5782, 4.4988) -> (17.6003, 4.5815)
  line L1564 (17.5177, 4.4383) -> (17.5782, 4.4988)
  line L1565 (17.435, 4.4161) -> (17.5177, 4.4383)
  line L1566 (17.2918, 4.4988) -> (17.3523, 4.4383)
  line L1567 (17.2697, 4.5815) -> (17.2918, 4.4988)
  line L1568 (17.2918, 4.6641) -> (17.2697, 4.5815)
  line L1569 (17.435, 4.7468) -> (17.3523, 4.7246)
  line L1570 (17.6003, 1.5272) -> (17.5782, 1.6098)
  line L1571 (17.5782, 1.4445) -> (17.6003, 1.5272)
  line L1572 (17.5177, 1.384) -> (17.5782, 1.4445)
  line L1573 (17.435, 1.3618) -> (17.5177, 1.384)
  line L1574 (17.3523, 1.384) -> (17.435, 1.3618)
  line L1575 (17.2918, 1.4445) -> (17.3523, 1.384)
  line L1576 (17.2697, 1.5272) -> (17.2918, 1.4445)
  line L1577 (17.2918, 1.6098) -> (17.2697, 1.5272)
  line L1578 (17.3523, 1.6703) -> (17.2918, 1.6098)
  line L1579 (17.435, 1.6925) -> (17.3523, 1.6703)
  line L1580 (17.5177, 1.6703) -> (17.435, 1.6925)
  line L1581 (17.5782, 1.6098) -> (17.5177, 1.6703)
  line L1582 (1.6925, 3.5634) -> (1.6703, 3.646)
  line L1583 (1.5272, 3.398) -> (1.6186, 3.4114)
  line L1584 (1.4445, 3.4202) -> (1.5272, 3.398)
  line L1585 (1.384, 3.4807) -> (1.4445, 3.4202)
  line L1586 (1.3618, 3.5634) -> (1.384, 3.4807)
  line L1587 (1.5272, 3.7287) -> (1.4445, 3.7065)
  line L1588 (1.6703, 3.646) -> (1.6098, 3.7065)
  line L1589 (5.2559, 0) -> (5.2337, 0.0827)
  line L1590 (5.2337, -0.0827) -> (5.2559, 0)
  line L1591 (5.1732, -0.1432) -> (5.2337, -0.0827)
  line L1592 (4.9473, -0.0827) -> (5.0078, -0.1432)
  line L1593 (4.9252, 0) -> (4.9473, -0.0827)
  line L1594 (4.9473, 0.0827) -> (4.9252, 0)
  line L1595 (5.0078, 0.1432) -> (4.9473, 0.0827)
  line L1596 (5.2337, 0.0827) -> (5.1732, 0.1432)
  line L1597 (3.3469, 1.7817) -> (3.3248, 1.8643)
  line L1598 (3.3248, 1.699) -> (3.3469, 1.7817)
  line L1599 (3.0989, 1.6385) -> (3.1816, 1.6163)
  line L1600 (3.0384, 1.699) -> (3.0989, 1.6385)
  line L1601 (3.0162, 1.7817) -> (3.0384, 1.699)
  line L1602 (3.0384, 1.8643) -> (3.0162, 1.7817)
  line L1603 (3.2642, 1.9249) -> (3.1816, 1.947)
  line L1604 (3.3248, 1.8643) -> (3.2642, 1.9249)
  line L1605 (16.3277, -9.1629) -> (16.3056, -9.0802)
  line L1606 (16.3056, -9.2456) -> (16.3277, -9.1629)
  line L1607 (16.245, -9.3061) -> (16.3056, -9.2456)
  line L1608 (16.1624, -9.3283) -> (16.245, -9.3061)
  line L1609 (16.0797, -9.3061) -> (16.1624, -9.3283)
  line L1610 (16.0192, -9.2456) -> (16.0797, -9.3061)
  line L1611 (15.997, -9.1629) -> (16.0192, -9.2456)
  line L1612 (16.0192, -9.0802) -> (15.997, -9.1629)
  line L1613 (16.0797, -9.0197) -> (16.0192, -9.0802)
  line L1614 (16.1502, -9.0008) -> (16.0797, -9.0197)
  line L1615 (16.245, -9.0197) -> (16.1502, -9.0008)
  line L1616 (16.3056, -9.0802) -> (16.245, -9.0197)
  line L1617 (2.7106, 16.0351) -> (2.6884, 16.1178)
  line L1618 (2.6884, 15.9524) -> (2.7106, 16.0351)
  line L1619 (2.5453, 15.8698) -> (2.6279, 15.8919)
  line L1620 (2.4626, 15.8919) -> (2.5453, 15.8698)
  line L1621 (2.4021, 15.9524) -> (2.4626, 15.8919)
  line L1622 (2.4021, 16.1178) -> (2.3799, 16.0351)
  line L1623 (2.4626, 16.1783) -> (2.4021, 16.1178)
  line L1624 (2.5453, 16.2004) -> (2.4626, 16.1783)
  line L1625 (2.6279, 16.1783) -> (2.5453, 16.2004)
  line L1626 (2.6884, 16.1178) -> (2.6279, 16.1783)
  line L1627 (7.1648, 15.9078) -> (7.1426, 15.9905)
  line L1628 (7.1426, 15.8252) -> (7.1648, 15.9078)
  line L1629 (7.0821, 15.7647) -> (7.1426, 15.8252)
  line L1630 (6.9995, 15.7425) -> (7.0821, 15.7647)
  line L1631 (6.9168, 15.7647) -> (6.9995, 15.7425)
  line L1632 (6.8563, 15.8252) -> (6.9168, 15.7647)
  line L1633 (6.8563, 15.9905) -> (6.8341, 15.9078)
  line L1634 (6.9168, 16.051) -> (6.8563, 15.9905)
  line L1635 (6.9995, 16.0732) -> (6.9168, 16.051)
  line L1636 (7.0821, 16.051) -> (6.9995, 16.0732)
  line L1637 (3.3469, 17.435) -> (3.3248, 17.5177)
  line L1638 (3.3248, 17.3523) -> (3.3469, 17.435)
  line L1639 (3.1816, 17.2697) -> (3.2642, 17.2918)
  line L1640 (3.0989, 17.2918) -> (3.1816, 17.2697)
  line L1641 (3.0384, 17.3523) -> (3.0989, 17.2918)
  line L1642 (3.0162, 17.435) -> (3.0384, 17.3523)
  line L1643 (3.0384, 17.5177) -> (3.0162, 17.435)
  line L1644 (3.0989, 17.5782) -> (3.0384, 17.5177)
  line L1645 (3.1816, 17.6003) -> (3.0989, 17.5782)
  line L1646 (3.2642, 17.5782) -> (3.1816, 17.6003)
  line L1647 (3.3248, 17.5177) -> (3.2642, 17.5782)
  line L1648 (-4.1616, 12.9808) -> (-4.1837, 13.0635)
  line L1649 (-4.1837, 12.8981) -> (-4.1616, 12.9808)
  line L1650 (-4.2443, 12.8376) -> (-4.1837, 12.8981)
  line L1651 (-4.3269, 12.8155) -> (-4.2443, 12.8376)
  line L1652 (-4.4096, 12.8376) -> (-4.3269, 12.8155)
  line L1653 (-4.4923, 12.9808) -> (-4.4701, 12.8981)
  line L1654 (-4.4701, 13.0635) -> (-4.4923, 12.9808)
  line L1655 (-4.4096, 13.124) -> (-4.4701, 13.0635)
  line L1656 (-4.3269, 13.1461) -> (-4.4096, 13.124)
  line L1657 (-4.2443, 13.124) -> (-4.3269, 13.1461)
  line L1658 (-4.1837, 13.0635) -> (-4.2443, 13.124)
  line L1659 (3.856, -2.1635) -> (3.8338, -2.0808)
  line L1660 (3.8338, -2.2461) -> (3.856, -2.1635)
  line L1661 (3.7733, -2.3067) -> (3.8338, -2.2461)
  line L1662 (3.6906, -2.3288) -> (3.7733, -2.3067)
  line L1663 (3.5253, -2.1635) -> (3.5474, -2.2461)
  line L1664 (3.5474, -2.0808) -> (3.5253, -2.1635)
  line L1665 (3.6079, -2.0203) -> (3.5474, -2.0808)
  line L1666 (3.6906, -1.9981) -> (3.6079, -2.0203)
  line L1667 (13.5279, -15.1443) -> (13.5058, -15.0616)
  line L1668 (13.5058, -15.2269) -> (13.5279, -15.1443)
  line L1669 (13.4453, -15.2875) -> (13.5058, -15.2269)
  line L1670 (13.3626, -15.3096) -> (13.4453, -15.2875)
  line L1671 (13.2799, -15.2875) -> (13.3626, -15.3096)
  line L1672 (13.2194, -15.2269) -> (13.2799, -15.2875)
  line L1673 (13.1972, -15.1443) -> (13.2194, -15.2269)
  line L1674 (13.2194, -15.0616) -> (13.1972, -15.1443)
  line L1675 (13.2799, -15.0011) -> (13.2194, -15.0616)
  line L1676 (13.3626, -14.9789) -> (13.2799, -15.0011)
  line L1677 (13.5058, -15.0616) -> (13.4453, -15.0011)
  line L1678 (-1.2345, 8.2721) -> (-1.2567, 8.3548)
  line L1679 (-1.2567, 8.1894) -> (-1.2345, 8.2721)
  line L1680 (-1.3172, 8.1289) -> (-1.2567, 8.1894)
  line L1681 (-1.3999, 8.1067) -> (-1.3172, 8.1289)
  line L1682 (-1.4826, 8.1289) -> (-1.3999, 8.1067)
  line L1683 (-1.5431, 8.1894) -> (-1.4826, 8.1289)
  line L1684 (-1.5652, 8.2721) -> (-1.5431, 8.1894)
  line L1685 (-1.5431, 8.3548) -> (-1.5652, 8.2721)
  line L1686 (-1.4826, 8.4153) -> (-1.5431, 8.3548)
  line L1687 (-1.3999, 8.4374) -> (-1.4826, 8.4153)
  line L1688 (-1.3172, 8.4153) -> (-1.3999, 8.4374)
  line L1689 (-1.2567, 8.3548) -> (-1.3172, 8.4153)
  line L1690 (-14.8517, 7.254) -> (-14.8738, 7.3366)
  line L1691 (-14.8738, 7.1713) -> (-14.8517, 7.254)
  line L1692 (-14.9343, 7.1108) -> (-14.8738, 7.1713)
  line L1693 (-15.017, 7.0886) -> (-14.9343, 7.1108)
  line L1694 (-15.0997, 7.1108) -> (-15.017, 7.0886)
  line L1695 (-15.1602, 7.1713) -> (-15.0997, 7.1108)
  line L1696 (-15.1823, 7.254) -> (-15.1602, 7.1713)
  line L1697 (-15.1602, 7.3366) -> (-15.1823, 7.254)
  line L1698 (-15.0997, 7.3972) -> (-15.1602, 7.3366)
  line L1699 (-15.017, 7.4193) -> (-15.0997, 7.3972)
  line L1700 (-14.9343, 7.3972) -> (-15.017, 7.4193)
  line L1701 (-14.8738, 7.3366) -> (-14.9343, 7.3972)
  line L1702 (-14.8517, 4.7087) -> (-14.8738, 4.7914)
  line L1703 (-14.8738, 4.6261) -> (-14.8517, 4.7087)
  line L1704 (-14.9343, 4.5655) -> (-14.8738, 4.6261)
  line L1705 (-15.0997, 4.5655) -> (-15.017, 4.5434)
  line L1706 (-15.1602, 4.6261) -> (-15.0997, 4.5655)
  line L1707 (-15.1823, 4.7087) -> (-15.1602, 4.6261)
  line L1708 (-15.1602, 4.7914) -> (-15.1823, 4.7087)
  line L1709 (-15.0997, 4.8519) -> (-15.1602, 4.7914)
  line L1710 (-15.017, 4.8741) -> (-15.0997, 4.8519)
  line L1711 (-14.9343, 4.8519) -> (-15.017, 4.8741)
  line L1712 (-15.2335, -0.6363) -> (-15.2556, -0.5536)
  line L1713 (-15.3161, -0.7795) -> (-15.2556, -0.719)
  line L1714 (-15.3988, -0.8017) -> (-15.3161, -0.7795)
  line L1715 (-15.4815, -0.7795) -> (-15.3988, -0.8017)
  line L1716 (-15.542, -0.719) -> (-15.4815, -0.7795)
  line L1717 (-15.5641, -0.6363) -> (-15.542, -0.719)
  line L1718 (-15.542, -0.5536) -> (-15.5641, -0.6363)
  line L1719 (-15.4815, -0.4931) -> (-15.542, -0.5536)
  line L1720 (-15.3988, -0.471) -> (-15.4815, -0.4931)
  line L1721 (-15.2556, -0.5536) -> (-15.3161, -0.4931)
  line L1722 (13.5279, 2.1635) -> (13.5058, 2.2461)
  line L1723 (13.5058, 2.0808) -> (13.5279, 2.1635)
  line L1724 (13.4453, 2.0203) -> (13.5058, 2.0808)
  line L1725 (13.3626, 1.9981) -> (13.4453, 2.0203)
  line L1726 (13.2194, 2.0808) -> (13.2799, 2.0203)
  line L1727 (13.2194, 2.2461) -> (13.1972, 2.1635)
  line L1728 (13.2799, 2.3067) -> (13.2194, 2.2461)
  line L1729 (13.3626, 2.3288) -> (13.2799, 2.3067)
  line L1730 (13.4453, 2.3067) -> (13.3626, 2.3288)
  line L1731 (13.5058, 2.2461) -> (13.4453, 2.3067)
  line L1732 (14.8006, 2.418) -> (14.7784, 2.5007)
  line L1733 (14.492, 2.3353) -> (14.5525, 2.2748)
  line L1734 (14.4699, 2.418) -> (14.492, 2.3353)
  line L1735 (14.492, 2.5007) -> (14.4699, 2.418)
  line L1736 (14.5525, 2.5612) -> (14.492, 2.5007)
  line L1737 (14.7179, 2.5612) -> (14.6352, 2.5833)
  line L1738 (-2.5898, 3.5474) -> (-2.5293, 3.6079)
  line L1739 (-2.8157, 3.7733) -> (-2.8379, 3.6906)
  line L1740 (-2.6725, 3.856) -> (-2.7552, 3.8338)
  line L1741 (-0.8082, 3.5474) -> (-0.7476, 3.6079)
  line L1742 (-0.8908, 3.5253) -> (-0.8082, 3.5474)
  line L1743 (-1.034, 3.7733) -> (-1.0562, 3.6906)
  line L1744 (-0.9735, 3.8338) -> (-1.034, 3.7733)
  line L1745 (-0.8908, 3.856) -> (-0.9735, 3.8338)
  line L1746 (-0.8082, 3.8338) -> (-0.8908, 3.856)
  line L1747 (-0.7476, 3.7733) -> (-0.8082, 3.8338)
  line L1748 (11.2372, -2.1635) -> (11.215, -2.0808)
  line L1749 (11.215, -2.2461) -> (11.2372, -2.1635)
  line L1750 (11.1545, -2.3067) -> (11.215, -2.2461)
  line L1751 (11.0719, -2.3288) -> (11.1545, -2.3067)
  line L1752 (10.9892, -2.3067) -> (11.0719, -2.3288)
  line L1753 (10.9287, -2.2461) -> (10.9892, -2.3067)
  line L1754 (10.9065, -2.1635) -> (10.9287, -2.2461)
  line L1755 (10.9287, -2.0808) -> (10.9065, -2.1635)
  line L1756 (10.9892, -2.0203) -> (10.9287, -2.0808)
  line L1757 (11.215, -2.0808) -> (11.1545, -2.0203)
  line L1758 (17.0691, 7.044) -> (17.0913, 7.1267)
  line L1759 (17.0086, 6.9835) -> (17.0691, 7.044)
  line L1760 (8.0176, 7.763) -> (7.9835, 7.8903)
  line L1761 (7.9835, 7.6358) -> (8.0176, 7.763)
  line L1762 (7.763, 7.5085) -> (7.8903, 7.5426)
  line L1763 (7.6358, 7.5426) -> (7.763, 7.5085)
  line L1764 (7.5426, 7.6358) -> (7.6358, 7.5426)
  line L1765 (7.5085, 7.763) -> (7.5426, 7.6358)
  line L1766 (7.5426, 7.8903) -> (7.5085, 7.763)
  line L1767 (7.763, 8.0176) -> (7.6358, 7.9835)
  line L1768 (7.8903, 7.9835) -> (7.763, 8.0176)
  line L1769 (7.9835, 7.8903) -> (7.8903, 7.9835)
  line L1770 (-7.5085, 7.763) -> (-7.5426, 7.8903)
  line L1771 (-7.5426, 7.6358) -> (-7.5085, 7.763)
  line L1772 (-7.763, 8.0176) -> (-7.8903, 7.9835)
  line L1773 (8.0176, -7.763) -> (7.9835, -7.6358)
  line L1774 (7.9835, -7.8903) -> (8.0176, -7.763)
  line L1775 (7.8903, -7.9835) -> (7.9835, -7.8903)
  line L1776 (7.763, -8.0176) -> (7.8903, -7.9835)
  line L1777 (7.6358, -7.9835) -> (7.763, -8.0176)
  line L1778 (7.5085, -7.763) -> (7.5426, -7.8903)
  line L1779 (7.5426, -7.6358) -> (7.5085, -7.763)
  line L1780 (7.6358, -7.5426) -> (7.5426, -7.6358)
  line L1781 (7.763, -7.5085) -> (7.6358, -7.5426)
  line L1782 (7.8903, -7.5426) -> (7.763, -7.5085)
  line L1783 (-8.0433, 18.2747) -> (-7.9701, 18.1449)
  line L1784 (18.1449, -8.2246) -> (18.2747, -8.2953)
  line L1785 (-13.5897, -17.1517) -> (-13.7258, -17.2743)
  line L1786 (-14.7716, 16.1624) -> (-14.9979, 16.3752)
  line L1787 (-14.9979, 16.3752) -> (-15.502, 16.5103)
  line L1788 (-15.502, 16.5103) -> (-16.0062, 16.3752)
  line L1789 (-16.0062, 16.3752) -> (-16.3752, 16.0062)
  line L1790 (-16.3752, 16.0062) -> (-16.5103, 15.502)
  line L1791 (-16.5103, 15.502) -> (-16.3752, 14.9979)
  line L1792 (-16.3752, 14.9979) -> (-16.1624, 14.7716)
  line L1793 (5.7885, 16.0062) -> (5.4194, 16.3752)
  line L1794 (5.4194, 16.3752) -> (4.9153, 16.5103)
  line L1795 (4.4111, 16.3752) -> (4.0421, 16.0062)
  line L1796 (4.0421, 16.0062) -> (3.9451, 15.6533)
  line L1797 (5.8449, 15.1443) -> (5.9235, 15.502)
  line L1798 (-16.6273, -14.9979) -> (-16.7624, -15.502)
  line L1799 (-16.7624, -15.502) -> (-16.6273, -16.0062)
  line L1800 (-16.6273, -16.0062) -> (-16.2582, -16.3752)
  line L1801 (-16.2582, -16.3752) -> (-15.7541, -16.5103)
  line L1802 (-15.7541, -16.5103) -> (-15.25, -16.3752)
  line L1803 (15.8711, -2.3946) -> (15.502, -2.0256)
  line L1804 (15.502, -2.0256) -> (15.1055, -1.9193)
  line L1805 (14.6352, -3.8087) -> (14.9979, -3.907)
  line L1806 (14.9979, -3.907) -> (15.502, -3.7719)
  line L1807 (15.502, -3.7719) -> (15.8711, -3.4029)
  line L1808 (15.8711, -3.4029) -> (16.0062, -2.8988)
  line L1809 (-13.1763, 15.2715) -> (-13.2334, 15.3085)
  line L1810 (-13.2334, 15.3085) -> (-13.4855, 15.376)
  line L1811 (-13.4855, 15.376) -> (-13.7376, 15.3085)
  line L1812 (-13.7376, 15.3085) -> (-13.9221, 15.1239)
  line L1813 (-13.9221, 15.1239) -> (-13.9896, 14.8719)
  line L1814 (-13.9896, 14.8719) -> (-13.9246, 14.6291)
  line L1815 (-13.9246, 14.6291) -> (-13.8716, 14.5762)
  line L1816 (-8.0567, 16.1813) -> (-8.1921, 16.3167)
  line L1817 (-8.1921, 16.3167) -> (-8.4442, 16.3843)
  line L1818 (-8.4442, 16.3843) -> (-8.6963, 16.3167)
  line L1819 (-8.6963, 16.3167) -> (-8.8808, 16.1322)
  line L1820 (-8.8808, 16.1322) -> (-8.9483, 15.8801)
  line L1821 (-8.9483, 15.8801) -> (-8.9049, 15.718)
  line L1822 (-8.0639, 14.172) -> (-8.1921, 14.3002)
  line L1823 (-8.6963, 14.3002) -> (-8.8808, 14.1157)
  line L1824 (-12.441, 13.1354) -> (-12.4772, 13.1451)
  line L1825 (-12.4772, 13.1451) -> (-12.5591, 13.1232)
  line L1826 (-12.5591, 13.1232) -> (-12.619, 13.0632)
  line L1827 (-12.619, 13.0632) -> (-12.641, 12.9814)
  line L1828 (-12.641, 12.9814) -> (-12.6331, 12.9518)
  line L1829 (-1.0524, 5.8133) -> (-1.1343, 5.8352)
  line L1830 (-1.1343, 5.8352) -> (-1.2162, 5.8133)
  line L1831 (-1.298, 5.6715) -> (-1.2886, 5.6442)
  line L1832 (-9.0901, 17.3484) -> (-9.1183, 17.2918)
  line L1833 (11.3807, 12.7293) -> (11.3587, 12.8112)
  line L1834 (11.3587, 12.8112) -> (11.2988, 12.8711)
  line L1835 (11.2988, 12.8711) -> (11.2169, 12.8931)
  line L1836 (11.2169, 12.8931) -> (11.1681, 12.88)
  line L1837 (11.373, 12.7007) -> (11.3807, 12.7293)
  line L1838 (-11.6701, 17.435) -> (-11.721, 17.4302)
  line L1839 (-11.8029, 17.4083) -> (-11.8629, 17.3484)
  line L1840 (-11.8629, 17.3484) -> (-11.8807, 17.2818)
  line L1841 (10.6025, 13.3153) -> (10.5426, 13.3752)
  line L1842 (10.5426, 13.3752) -> (10.4607, 13.3972)
  line L1843 (10.4607, 13.3972) -> (10.3975, 13.3626)
  line L1844 (10.6188, 13.2122) -> (10.6245, 13.2334)
  line L1845 (8.1002, 15.0011) -> (8.0819, 15.0798)
  line L1846 (8.0819, 15.0798) -> (8.0219, 15.1397)
  line L1847 (8.0219, 15.1397) -> (7.9401, 15.1616)
  line L1848 (7.9401, 15.1616) -> (7.8522, 15.1443)
  line L1849 (-1.3045, 16.4) -> (-1.3864, 16.422)
  line L1850 (-1.3864, 16.422) -> (-1.4682, 16.4)
  line L1851 (-1.4682, 16.4) -> (-1.5431, 16.3342)
  line L1852 (10.6245, 15.25) -> (10.6025, 15.3318)
  line L1853 (10.6025, 15.3318) -> (10.5426, 15.3918)
  line L1854 (17.4302, 7.9401) -> (17.4083, 8.0219)
  line L1855 (17.4083, 8.0219) -> (17.3484, 8.0819)
  line L1856 (17.3484, 8.0819) -> (17.2918, 8.1002)
  line L1857 (17.4086, 7.8593) -> (17.4302, 7.9401)
  line L1858 (14.4054, -12.4772) -> (14.3807, -12.4337)
  line L1859 (14.2417, -12.641) -> (14.3236, -12.619)
  line L1860 (14.3236, -12.619) -> (14.3835, -12.5591)